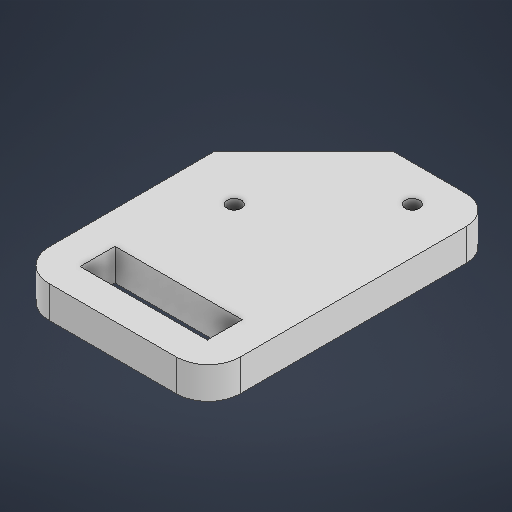
# Autodesk Inventor part: hip hitam
Saved by Autodesk Inventor 2026.2 (Build 302298010, 298A)
## iProperties
Created: 2026-05-10
Part Number: hip hitam
Material: Generic
Document SubType Name: Modeling
Designer: Martina
Density: 1 g/cm^3
Appearance: Default
Author: Martina
Autodesk Inventor part; units mm, degrees
ref_plane "YZ Plane" through (0, 0, 0) normal (1, 0, 0) x (0, 1, 0)
ref_plane "XZ Plane" through (0, 0, 0) normal (0, 1, 0) x (-1, 0, 0)
ref_plane "XY Plane" through (0, 0, 0) normal (0, 0, 1) x (1, 0, 0)
sketch "Sketch1" plane through (0, 0, 0) normal (0, 1, 0) x (-1, 0, 0)
  line L0 (-20.151, 40.9405) -> (15.849, 40.9405)
  line L1 (24.849, 31.9405) -> (24.849, -14.8595)
  line L2 (-0.351, -40.0595) -> (-21.051, -40.0595)
  line L3 (-29.151, -31.9595) -> (-29.151, 31.9405)
  arc A0 (24.849, 31.9405) -> (15.849, 40.9405) centre (15.849, 31.9405) ccw
  arc A1 (-20.151, 40.9405) -> (-29.151, 31.9405) centre (-20.151, 31.9405) ccw
  arc A2 (-29.151, -31.9595) -> (-21.051, -40.0595) centre (-21.051, -31.9595) ccw
  line L4 (24.849, -14.8595) -> (-0.351, -40.0595)
  circle A3 centre (9.082, -4.6389) radius 2.03
  circle A4 centre (-16.112, -29.8255) radius 2.03
  line L5 (15.664, 32.3905) -> (-20.336, 32.3905)
  line L6 (-20.336, 32.3905) -> (-20.336, 22.4905)
  line L7 (-20.336, 22.4905) -> (15.664, 22.4905)
  line L8 (15.664, 22.4905) -> (15.664, 32.3905)
  point P0 (0, 0)
  point P1 (-29.151, 40.9405)
  point P2 (24.849, -40.0595)
  point P3 (24.849, 40.9405)
  point P4 (-29.151, -40.0595)
  dimension "d0" = 9
  dimension "d1" = 8.1
  dimension "d2" = 20.7
  dimension "d3" = 36
  dimension "d4" = 46.8
  dimension "d5" = 9
  dimension "d6" = 63.9
  dimension "d7" = 4.06
  dimension "d8" = 4.06
  dimension "d9" = 15.767
  dimension "d10" = 18.376
  dimension "d11" = 10.234
  dimension "d12" = 13.039
  dimension "d13" = 38.233
  dimension "d14" = 9.9
  dimension "d15" = 36
  dimension "d16" = 8.55
  dimension "d17" = 8.815
  dimension "d18" = 9.185
  constraints: 18 end point, 8 point on line, 6 point on circle, 6 tangent, 5 centre point, 4 parallel, 2 horizontal, 2 perpendicular, 1 equal radius
  measures "d0" radius of A0
  measures "d1" radius of A2
  measures "d2" distance of L4.end L2.end
  measures "d3" distance of L0.start L0.end
  measures "d4" distance of L1.start L1.end
  measures "d5" radius of A1
  measures "d6" distance of L3.start L3.end
  measures "d7" diameter of A3
  measures "d8" diameter of A4
  measures "d9" distance from line of A3.centre L1
  measures "d10" distance from line of L4 A3.centre
  measures "d11" distance from line of L2 A4.centre
  measures "d12" distance from line of L3 A4.centre
  measures "d13" distance from line of L3 A3.centre
  measures "d14" distance of L8.start L5.start
  measures "d15" distance of L6.end L8.start
  measures "d16" distance between parallel lines of L5 L0
  measures "d17" distance between parallel lines of L3 L6
  measures "d18" distance between parallel lines of L8 L1
extrude "Extrusion1" add sketch "Sketch1" along normal blind 9
body "Solid1"
